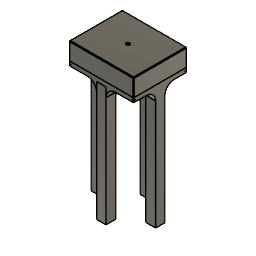
sensing_box (アセンブリ) (Autodesk Fusion 360 archive; units mm, degrees)
design "sensing_box"
Autodesk Fusion 360 part; units mm, degrees
sketch "スケッチ1" plane through (0, 0, 0) normal (0, 0, 1) x (1, 0, 0)
  line L0 (50, 40) -> (-50, 40)
  line L1 (-50, 40) -> (-50, -40)
  line L2 (-50, -40) -> (50, -40)
  line L3 (50, -40) -> (50, 40)
  line L4 (50, 40) -> (-50, -40) construction
  line L5 (-50, 40) -> (50, -40) construction
  line L6 (-46, 27.5) -> (20.5, 27.5)
  line L7 (20.5, 27.5) -> (20.5, -27.5)
  line L8 (20.5, -27.5) -> (-46, -27.5)
  line L9 (-46, -27.5) -> (-46, 27.5)
  line L10 (-46, 27.5) -> (20.5, -27.5) construction
  line L11 (20.5, 27.5) -> (-46, -27.5) construction
  line L12 (-50, 0) -> (-46, 0)
  line L13 (-46, 27.5) -> (-43.75, 27.5)
  line L14 (-43.75, 27.5) -> (-43.75, 25.25)
  line L15 (-43.75, 25.25) -> (-46, 25.25)
  line L16 (-46, 25.25) -> (-46, 27.5)
  line L17 (20, 0) -> (2.5, 0)
  line L18 (-43.75, -27.5) -> (-43.75, -25.25)
  line L19 (-43.75, -25.25) -> (-46, -25.25)
  line L20 (-12.75, 27.5) -> (-12.75, 25)
  line L21 (18.25, 25.25) -> (20.5, 25.25)
  line L22 (18.25, 27.5) -> (18.25, 25.25)
  line L23 (18.25, -25.25) -> (20.5, -25.25)
  line L24 (18.25, -27.5) -> (18.25, -25.25)
  line L25 (47.5, 27) -> (23.5, 27)
  line L26 (23.5, 27) -> (23.5, -27)
  line L27 (23.5, -27) -> (47.5, -27)
  line L28 (47.5, -27) -> (47.5, 27)
  line L29 (47.5, 27) -> (23.5, -27) construction
  line L30 (23.5, 27) -> (47.5, -27) construction
  line L31 (20.5, 0) -> (23.5, 0)
  line L32 (47.5, 27) -> (45, 27)
  line L33 (45, 27) -> (45, 18)
  line L34 (45, 18) -> (47.5, 18)
  line L35 (47.5, 18) -> (47.5, 27)
  line L36 (23.5, -27) -> (26, -27)
  line L37 (26, -27) -> (26, -18)
  line L38 (26, -18) -> (23.5, -18)
  line L39 (23.5, -18) -> (23.5, -27)
  point P0 (-12.75, 0)
  point P1 (35.5, 0)
  dimension "d1" = 100
  dimension "d2" = 80
  dimension "d3" = 66.5
  dimension "d4" = 55
  dimension "d5" = 4
  dimension "d6" = 2.25
  dimension "d7" = 2.25
  dimension "d8" = 24
  dimension "d9" = 54
  dimension "d10" = 3
  dimension "d13" = 2.5
  dimension "d14" = 9
  dimension "d15" = 2.5
  dimension "d16" = 9
  constraint horizontal L0
  constraint perpendicular L0 L1
  constraint parallel L0 L2
  constraint parallel L1 L3
  constraint coincident L4 origin
  constraint coincident L5 origin
  constraint horizontal L6
  constraint perpendicular L6 L7
  constraint parallel L6 L8
  constraint parallel L7 L9
  constraint coincident L10 P0
  constraint coincident L11 P0
  constraint midpoint L1 L12.start
  constraint midpoint L9 L12.end
  constraint perpendicular L9 L12
  constraint horizontal L13
  constraint vertical L14
  constraint horizontal L15
  constraint vertical L16
  constraint symmetric L13.end L17 L18.start
  constraint symmetric L14.end L17 L18.end
  constraint symmetric L15.end L17 L19.end
  constraint midpoint L6 L20.start
  constraint perpendicular L6 L20
  constraint symmetric L13.end L20 L22.start
  constraint symmetric L14.end L20 L21.start
  constraint symmetric L15.end L20 L21.end
  constraint symmetric L18.start L20 L24.start
  constraint symmetric L18.end L20 L23.start
  constraint symmetric L19.end L20 L23.end
  constraint horizontal L25
  constraint perpendicular L25 L26
  constraint parallel L25 L27
  constraint parallel L26 L28
  constraint coincident L29 P1
  constraint coincident L30 P1
  constraint midpoint L7 L31.start
  constraint midpoint L26 L31.end
  constraint horizontal L32
  constraint vertical L33
  constraint horizontal L34
  constraint vertical L35
  constraint horizontal L36
  constraint vertical L37
  constraint horizontal L38
  constraint vertical L39
  measures "d1" distance of L1.end L2.end
  measures "d2" distance of L0.end L1.end
  measures "d3" distance of L7.end L8.end
  measures "d4" distance of L6.end L7.end
  measures "d5" distance of L12.start L12.end
  measures "d6" distance of L6.start L13.end
  measures "d7" distance of L6.start L15.end
  measures "d8" distance of L26.end L27.end
  measures "d9" distance of L25.end L26.end
  measures "d10" distance of L31.start L31.end
  measures "d13" distance of L25.start L32.end
  measures "d14" distance of L25.start L34.end
  measures "d15" distance of L26.end L36.end
  measures "d16" distance of L26.end L38.end
extrude "押し出し1" add sketch "スケッチ1" along normal blind 5 makes body 1
extrude "押し出し2" add sketch "スケッチ1" along normal blind 3.5 contours L6 L9 L13 L14 L15 L16 | L6 L7 L8 L9 L14 L15 L18 L19 L21 L22 L23 L24 | L6 L7 L21 L22 | L8 L9 L18 L19 | L7 L8 L23 L24 | L25 L28 L32 L33 L34 L35 | L25 L26 L27 L28 L33 L34 L37 L38 | L26 L27 L36 L37 L38 L39 bodies 1
extrude "押し出し3" add sketch "スケッチ1" against normal blind 2 contours L0 L1 L2 L3 | L6 L9 L13 L14 L15 L16 | L6 L7 L8 L9 L14 L15 L18 L19 L21 L22 L23 L24 | L6 L7 L21 L22 | L8 L9 L18 L19 | L7 L8 L23 L24 | L25 L28 L32 L33 L34 L35 | L25 L26 L27 L28 L33 L34 L37 L38 | L26 L27 L36 L37 L38 L39 bodies 1
sketch "スケッチ2" plane through (0, 0, 3.5) normal (0, 0, 1) x (-1, 0, 0)
  line L0 (-23.5, -27) -> (-23.5, 27)
  line L1 (-23.5, 27) -> (-47.5, 27)
  line L2 (-47.5, 27) -> (-47.5, -27)
  line L3 (-47.5, -27) -> (-23.5, -27)
  line L4 (-47.5, -27) -> (-45, -27)
  line L5 (-45, -27) -> (-45, -17.5)
  line L6 (-45, -17.5) -> (-47.5, -17.5)
  line L7 (-47.5, -17.5) -> (-47.5, -27)
  line L8 (-26, 16.5) -> (-23.5, 16.5)
  line L9 (-23.5, 16.5) -> (-23.5, 27)
  line L10 (-23.5, 27) -> (-26, 27)
  line L11 (-26, 27) -> (-26, 16.5)
  dimension "d90" = 10.5
  dimension "d103" = 9.5
  dimension "d104" = 2.5
  dimension "d105" = 2.5
  constraint horizontal L4
  constraint vertical L5
  constraint horizontal L6
  constraint vertical L7
  constraint coincident L2.end L3.start
  constraint horizontal L8
  constraint vertical L9
  constraint horizontal L10
  constraint vertical L11
  constraint coincident L0.end L1.start
  measures "d90" distance of L8.start L10.end
  measures "d103" distance of L4.end L5.end
  measures "d104" distance of L5.end L6.end
  measures "d105" distance of L8.start L8.end
sketch "スケッチ3" plane through (0, 0, 3.5) normal (0, 0, 1) x (-1, 0, 0)
  line L0 (46, -27.5) -> (46, 27.5)
  line L1 (46, 27.5) -> (-20.5, 27.5)
  line L2 (-20.5, 27.5) -> (-20.5, -27.5)
  line L3 (-20.5, -27.5) -> (46, -27.5)
  line L4 (-20.5, 27.5) -> (-17.75, 27.5)
  line L5 (-17.75, 27.5) -> (-17.75, 24.75)
  line L6 (-17.75, 24.75) -> (-20.5, 24.75)
  line L7 (-20.5, 24.75) -> (-20.5, 27.5)
  line L8 (46, 27.5) -> (43.25, 27.5)
  line L9 (43.25, 27.5) -> (43.25, 24.75)
  line L10 (43.25, 24.75) -> (46, 24.75)
  line L11 (46, 24.75) -> (46, 27.5)
  line L12 (-20, 0) -> (-2.5, 0)
  line L13 (-17.75, -24.75) -> (-20.5, -24.75)
  line L14 (-17.75, -27.5) -> (-17.75, -24.75)
  line L15 (43.25, -27.5) -> (43.25, -24.75)
  line L16 (43.25, -24.75) -> (46, -24.75)
  dimension "d21" = 2.75
  dimension "d22" = 2.75
  dimension "d23" = 2.75
  dimension "d24" = 2.75
  constraint horizontal L4
  constraint vertical L5
  constraint horizontal L6
  constraint vertical L7
  constraint coincident L1.end L2.start
  constraint horizontal L8
  constraint vertical L9
  constraint horizontal L10
  constraint vertical L11
  constraint coincident L0.end L1.start
  constraint symmetric L4.end L12 L14.start
  constraint symmetric L5.end L12 L13.start
  constraint symmetric L6.end L12 L13.end
  constraint symmetric L8.end L12 L15.start
  constraint symmetric L9.end L12 L15.end
  constraint symmetric L10.end L12 L16.end
  measures "d21" distance of L1.end L4.end
  measures "d22" distance of L1.end L6.end
  measures "d23" distance of L0.end L8.end
  measures "d24" distance of L0.end L10.end
hole "穴1" at (45, 17.5, 3.5) at (26, -16.5, 3.5) at (17.75, 24.75, 3.5) at (17.75, -24.75, 3.5) at (-43.25, 24.75, 3.5) at (-43.25, -24.75, 3.5) direction (0, 0, -1) diameter 2.529 depth 5 tip angle 180 bodies 1
thread "ねじ1" "ISO Metric profile 3.0 M3x0.5 M3x0.5 6H" thread offset 0 thread depth 7.4
sketch "スケッチ4" plane through (0, 0, 5) normal (0, 0, 1) x (-1, 0, 0)
  line L0 (46, 27.5) -> (46, -27.5)
  line L1 (46, -27.5) -> (-20.5, -27.5)
  line L2 (-20.5, -27.5) -> (-20.5, 27.5)
  line L3 (-20.5, 27.5) -> (46, 27.5)
  line L4 (-47.5, -27) -> (-47.5, 27)
  line L5 (-47.5, 27) -> (-23.5, 27)
  line L6 (-23.5, 27) -> (-23.5, -27)
  line L7 (-23.5, -27) -> (-47.5, -27)
  line L8 (-50, 40) -> (-50, -40)
  line L9 (-50, -40) -> (50, -40)
  line L10 (50, -40) -> (50, 40)
  line L11 (50, 40) -> (-50, 40)
  circle A0 centre (-19.9469, -38.0053) radius 4.5
  line L12 (32.5531, -28.2121) -> (7.5531, -28.2121)
  line L13 (7.5531, -28.2121) -> (7.5531, -47.7121)
  line L14 (7.5531, -47.7121) -> (32.5531, -47.7121)
  line L15 (32.5531, -47.7121) -> (32.5531, -28.2121)
  line L16 (32.5531, -28.2121) -> (7.5531, -47.7121) construction
  line L17 (7.5531, -28.2121) -> (32.5531, -47.7121) construction
  line L18 (32.5531, -28.2121) -> (7.5531, -28.2121)
  line L19 (7.5531, -28.2121) -> (7.5531, -31.2121)
  line L20 (7.5531, -31.2121) -> (32.5531, -31.2121)
  line L21 (32.5531, -31.2121) -> (32.5531, -28.2121)
  line L22 (32.5531, -47.7121) -> (30.0531, -47.7121)
  line L23 (30.0531, -47.7121) -> (30.0531, -45.2121)
  line L24 (30.0531, -45.2121) -> (32.5531, -45.2121)
  line L25 (32.5531, -45.2121) -> (32.5531, -47.7121)
  line L26 (20.0531, -37.9621) -> (0.0531, -37.9621)
  line L27 (0.0531, -37.9621) -> (-19.9469, -38.0053)
  line L28 (20.0531, -47.7121) -> (20.0531, -43)
  line L29 (10.0531, -47.7121) -> (10.0531, -45.2121)
  line L30 (10.0531, -45.2121) -> (7.5531, -45.2121)
  point P0 (20.0531, -37.9621)
  dimension "d30" = 9
  dimension "d31" = 25
  dimension "d32" = 19.5
  dimension "d33" = 3
  dimension "d34" = 2.5
  dimension "d35" = 2.5
  dimension "d40" = 20
  dimension "d41" = 20
  constraint horizontal L12
  constraint perpendicular L12 L13
  constraint parallel L12 L14
  constraint parallel L13 L15
  constraint coincident L16 P0
  constraint coincident L17 P0
  constraint horizontal L18
  constraint vertical L19
  constraint horizontal L20
  constraint vertical L21
  constraint coincident L13 L19.end
  constraint horizontal L22
  constraint vertical L23
  constraint horizontal L24
  constraint vertical L25
  constraint coincident P0 L26.start
  constraint perpendicular L13 L26
  constraint coincident A0.centre L27.end
  constraint midpoint L14 L28.start
  constraint perpendicular L14 L28
  constraint symmetric L22.end L28 L29.start
  constraint symmetric L23.end L28 L29.end
  constraint symmetric L24.end L28 L30.end
  measures "d30" diameter of A0
  measures "d31" distance of L13.end L14.end
  measures "d32" distance of L12.end L13.end
  measures "d33" distance of L12.start L20.end
  measures "d34" distance of L14.end L22.end
  measures "d35" distance of L14.end L24.end
  measures "d40" distance of P0 L26.end
  measures "d41" horizontal distance of L26.end A0.centre
extrude "押し出し4" cut 1 faces at (16.6667, -40, 0.3333) along direction (0, 1, 0) blind 8.25 on bodies 1 bodies 1
extrude "押し出し5" add 1 faces at (16.6667, 40, 2.6667) along direction (0, 1, 0) blind 10.25 on bodies 1 bodies 1
extrude "押し出し6" cut sketch "スケッチ4" against normal blind 7 contours L9 A0 | L9 A0 | L12 L13 L15 L18 L19 L20 L21 bodies 1
extrude "押し出し7" cut sketch "スケッチ4" along normal blind 2 from surface at -7 contours L9 L13 L14 L15 L23 L24 L29 L30 | L9 L13 L15 L20 | L14 L15 L22 L23 L24 L25 | L13 L14 L29 L30 bodies 1
hole "穴2" at (-10.0531, 45.2121, 5) direction (0, 0, -1) diameter 2.529 end up to surface (7 mm away) bodies 1
thread "ねじ2" "ISO Metric profile 3.0 M3x0.5 M3x0.5 6H" major diameter 3.086 minor diameter 2.529 pitch 0.5 angle 60 resizes the face on face at (-11.3172, 45.2436, 3.3333) on bodies 1
extrude "押し出し8" add 1 faces at (16.6667, 50.25, 2.6667) along direction (0, 1, 0) blind 2 on bodies 1 bodies 1
extrude "押し出し9" add 1 faces at (-50, 24.25, 0.3333) along direction (-1, 0, 0) blind 2 on bodies 1 bodies 1
extrude "押し出し10" add 1 faces at (16, -31.75, 2.6667) along direction (0, -1, 0) blind 2 on bodies 1 bodies 1
extrude "押し出し11" add 1 faces at (50, -5.0833, 2.6667) along direction (1, 0, 0) blind 2 on bodies 1 bodies 1
sketch "スケッチ5" plane through (0, 0, 5) normal (0, 0, 1) x (-1, 0, 0)
  line L0 (7.5531, -28.2121) -> (32.5531, -28.2121)
  line L1 (32.5531, -28.2121) -> (32.5531, -31.2121)
  line L2 (32.5531, -31.2121) -> (7.5531, -31.2121)
  line L3 (7.5531, -31.2121) -> (7.5531, -28.2121)
  circle A0 centre (-19.9469, -38.0053) radius 4.5
  line L4 (-52, -52.25) -> (52, -52.25)
  line L5 (52, -52.25) -> (52, 33.75)
  line L6 (52, 33.75) -> (-52, 33.75)
  line L7 (-52, 33.75) -> (-52, -52.25)
  line L8 (46, 27.5) -> (46, -27.5)
  line L9 (46, -27.5) -> (-20.5, -27.5)
  line L10 (-20.5, -27.5) -> (-20.5, 27.5)
  line L11 (-20.5, 27.5) -> (46, 27.5)
  line L12 (-47.5, -27) -> (-47.5, 27)
  line L13 (-47.5, 27) -> (-23.5, 27)
  line L14 (-23.5, 27) -> (-23.5, -27)
  line L15 (-23.5, -27) -> (-47.5, -27)
  line L16 (-47, 28.75) -> (47, 28.75)
  line L17 (47, 28.75) -> (47, -47.25)
  line L18 (47, -47.25) -> (-47, -47.25)
  line L19 (-47, -47.25) -> (-47, 28.75)
  line L20 (-47, 28.75) -> (47, -47.25) construction
  line L21 (47, 28.75) -> (-47, -47.25) construction
  circle A1 centre (10.0531, -45.2121) radius 1.2645
  point P0 (0, -9.25)
  dimension "d59" = 94
  dimension "d60" = 76
  constraint horizontal L16
  constraint perpendicular L16 L17
  constraint parallel L16 L18
  constraint parallel L17 L19
  constraint coincident L20 P0
  constraint coincident L21 P0
  measures "d59" distance of L17.end L18.end
  measures "d60" distance of L16.end L17.end
extrude "押し出し12" add sketch "スケッチ5" along normal blind 25 contours L4 L5 L6 L7 | L12 L13 L15 L19 bodies 1
sketch "スケッチ6" plane through (0, 0, -2) normal (0, 0, -1) x (1, 0, 0)
  line L0 (-52, 33.75) -> (-52, -52.25)
  line L1 (-52, -52.25) -> (52, -52.25)
  line L2 (52, -52.25) -> (52, 33.75)
  line L3 (52, 33.75) -> (-52, 33.75)
  circle A0 centre (19.9469, -38.0053) radius 4.5
  line L4 (-7.5531, -28.2121) -> (-7.5531, -47.7121)
  line L5 (-7.5531, -47.7121) -> (-32.5531, -47.7121)
  line L6 (-32.5531, -47.7121) -> (-32.5531, -28.2121)
  line L7 (-32.5531, -28.2121) -> (-7.5531, -28.2121)
  line L8 (-52, 33.75) -> (-49, 33.75)
  line L9 (-49, 33.75) -> (-49, 30.75)
  line L10 (-49, 30.75) -> (-52, 30.75)
  line L11 (-52, 30.75) -> (-52, 33.75)
  line L12 (-52, -52.25) -> (-49, -52.25)
  line L13 (-49, -52.25) -> (-49, -49.25)
  line L14 (-49, -49.25) -> (-52, -49.25)
  line L15 (-52, -49.25) -> (-52, -52.25)
  line L16 (0, -1.75) -> (0, -22.5)
  line L17 (49, 30.75) -> (52, 30.75)
  line L18 (49, 33.75) -> (49, 30.75)
  line L19 (49, -49.25) -> (52, -49.25)
  line L20 (49, -52.25) -> (49, -49.25)
  dimension "d63" = 3
  dimension "d64" = 3
  dimension "d65" = 3
  dimension "d66" = 3
  constraint horizontal L8
  constraint vertical L9
  constraint horizontal L10
  constraint vertical L11
  constraint coincident L0.start L3.end
  constraint horizontal L12
  constraint vertical L13
  constraint horizontal L14
  constraint vertical L15
  constraint coincident L0.end L1.start
  constraint symmetric L8.end L16 L18.start
  constraint symmetric L9.end L16 L17.start
  constraint symmetric L10.end L16 L17.end
  constraint symmetric L12.end L16 L20.start
  constraint symmetric L13.end L16 L19.start
  constraint symmetric L14.end L16 L19.end
  measures "d63" distance of L0.start L8.end
  measures "d64" distance of L0.start L10.end
  measures "d65" distance of L0.end L12.end
  measures "d66" distance of L0.end L14.end
hole "穴3" at (-49, -30.75, -2) at (49, -30.75, -2) at (49, 49.25, -2) at (-49, 49.25, -2) direction (0, 0, 1) diameter 2.93 depth 15 tip angle 180 counterbore diameter 5 counterbore depth 3 bodies 1
thread "ねじ3" "ISO Metric profile 3.5 M3.5x0.6 M3.5x0.6 6H" major diameter 3.5995 minor diameter 2.93 pitch 0.6 angle 60 resizes the face on face at (-47.9016, 48.2806, 5) on face at (48.2994, -32.0366, 5) on face at (-49.7006, -32.0366, 5) on face at (50.0984, 48.2806, 5) on bodies 1
ref_plane "作業平面1" through (0, 9.25, 5) normal (0, 0, 1) x (1, 0, 0)
split "分割1" by plane through (0, 9.25, 5) normal (0, 0, 1) bodies 1 makes body 2 at (-17.3333, -33.75, 13.3333)
sketch "スケッチ7" plane through (0, 0, 30) normal (0, 0, 1) x (-1, 0, 0)
  line L0 (47, -47.25) -> (-47, -47.25)
  line L1 (-47, -47.25) -> (-47, 28.75)
  line L2 (-47, 28.75) -> (47, 28.75)
  line L3 (47, 28.75) -> (47, -47.25)
  line L4 (-52, 33.75) -> (-52, -52.25)
  line L5 (-52, -52.25) -> (52, -52.25)
  line L6 (52, -52.25) -> (52, 33.75)
  line L7 (52, 33.75) -> (-52, 33.75)
  line L8 (52, -52.25) -> (-52, -52.25)
  line L9 (-52, -52.25) -> (-52, 33.75)
  line L10 (-52, 33.75) -> (52, 33.75)
  line L11 (52, 33.75) -> (52, -52.25)
  constraint horizontal L8
  constraint vertical L9
  constraint horizontal L10
  constraint vertical L11
  constraint coincident L4.start L7.end
  constraint coincident L5.end L6.start
extrude "押し出し13" add sketch "スケッチ7" along normal blind 3 contours L0 L1 L2 L3 | L4 L5 L6 L7 L8 L9 L10 L11 bodies 2
sketch "スケッチ8" plane through (0, 0, 33) normal (0, 0, 1) x (-1, 0, 0)
  line L0 (52, 33.75) -> (-52, 33.75)
  line L1 (-52, 33.75) -> (-52, -52.25)
  line L2 (-52, -52.25) -> (52, -52.25)
  line L3 (52, -52.25) -> (52, 33.75)
  line L4 (52, -9.25) -> (-52, -9.25)
  ellipse E0 centre (0, -9.25) end of major axis (3, -9.25) minor radius 2.5
  line L5 (-3, -9.25) -> (3, -9.25) construction
  line L6 (0, -11.75) -> (0, -6.75) construction
  circle A0 centre (-1.5, -9.25) radius 0.75
  circle A1 centre (1.5, -9.25) radius 0.75
  dimension "d77" = 6
  dimension "d78" = 5
  dimension "d93" = 1.5
  dimension "d94" = 1.5
  dimension "d95" = 1.5
  dimension "d96" = 1.5
  constraint midpoint L3 L4.start
  constraint midpoint L1 L4.end
  constraint coincident E0 L5.start
  constraint coincident E0 L5.end
  constraint coincident E0 L6.start
  constraint coincident E0 L6.end
  constraint midpoint L4 E0.centre
  constraint perpendicular L3 L5
  constraint coincident L5 A0.centre
  constraint coincident L5 A1.centre
  measures "d77" distance of E0
  measures "d93" diameter of A0
  measures "d94" diameter of A1
  measures "d95" distance of E0.centre A0.centre
  measures "d96" distance of E0.centre A1.centre
extrude "押し出し14" cut sketch "スケッチ8" against normal blind 2 contours L4 E0 A0 A1 | L4 E0 A0 A1 | L4 A1 | L4 A1 | L4 A0 | L4 A0 bodies 2
sketch "スケッチ9" plane through (0, 52.25, 0) normal (0, 1, 0) x (-1, 0, 0)
  line L0 (-52, 5) -> (52, 5)
  line L1 (52, 5) -> (52, 33)
  line L2 (52, 33) -> (-52, 33)
  line L3 (-52, 33) -> (-52, 5)
  line L4 (-20.5, 31) -> (20.5, 31)
  line L5 (20.5, 31) -> (20.5, 15)
  line L6 (20.5, 15) -> (-20.5, 15)
  line L7 (-20.5, 15) -> (-20.5, 31)
  line L8 (-20.5, 31) -> (20.5, 15) construction
  line L9 (20.5, 31) -> (-20.5, 15) construction
  point P0 (0, 23)
  dimension "d84" = 41
  dimension "d85" = 16
  dimension "d86" = 10
  constraint horizontal L4
  constraint perpendicular L4 L5
  constraint parallel L4 L6
  constraint parallel L5 L7
  constraint coincident L8 P0
  constraint coincident L9 P0
  constraint vertical origin P0
  measures "d84" distance of L5.end L6.end
  measures "d85" distance of L4.end L5.end
  measures "d86" distance of L2 P0
extrude "押し出し15" cut sketch "スケッチ9" against normal up to surface (5 mm away) contours L4 L5 L6 L7 bodies 2
extrude "押し出し16" cut 1 faces at (-2.9129, -7.9872, 3.5) along direction (0, 0, -1) blind 1.5 on bodies 1 bodies 1
extrude "押し出し17" cut sketch "スケッチ8" against normal up to surface (3 mm away) contours L4 A1 | L4 A1 | L4 A0 | L4 A0 bodies 2
fillet "フィレット1" radius 1 8 edges at (52, -33.75, 1.5) (52, 9.25, -2) (52, 52.25, 1.5) (0, 52.25, -2) (-52, 52.25, 1.5) (-52, -33.75, 1.5) (-52, 9.25, -2) (0, -33.75, -2) on bodies 1
fillet "フィレット2" radius 1 8 edges at (52, -33.75, 19) (52, 9.25, 33) (0, -33.75, 33) (-52, 9.25, 33) (-52, -33.75, 19) (0, 52.25, 33) (-52, 52.25, 19) (52, 52.25, 19) on bodies 2
sketch "スケッチ10" plane through (0, 0, -2) normal (0, 0, -1) x (1, 0, 0)
  line L0 (-51, 29.25) -> (-51, -47.75)
  arc A0 (-47.5, -51.25) -> (-51, -47.75) centre (-49, -49.25) ccw
  line L1 (-47.5, -51.25) -> (47.5, -51.25)
  arc A1 (51, -47.75) -> (47.5, -51.25) centre (49, -49.25) ccw
  line L2 (51, -47.75) -> (51, 29.25)
  arc A2 (47.5, 32.75) -> (51, 29.25) centre (49, 30.75) ccw
  line L3 (47.5, 32.75) -> (-47.5, 32.75)
  arc A3 (-51, 29.25) -> (-47.5, 32.75) centre (-49, 30.75) ccw
  circle A4 centre (19.9469, -38.0053) radius 4.5
  line L4 (-7.5531, -28.2121) -> (-7.5531, -47.7121)
  line L5 (-7.5531, -47.7121) -> (-32.5531, -47.7121)
  line L6 (-32.5531, -47.7121) -> (-32.5531, -28.2121)
  line L7 (-32.5531, -28.2121) -> (-7.5531, -28.2121)
  line L8 (-66, -1.75) -> (-36, -1.75)
  line L9 (-36, -1.75) -> (-36, -16.75)
  line L10 (-36, -16.75) -> (-66, -16.75)
  line L11 (-66, -16.75) -> (-66, -1.75)
  line L12 (-66, -1.75) -> (-36, -16.75) construction
  line L13 (-36, -1.75) -> (-66, -16.75) construction
  line L14 (0, -1.75) -> (0, -22.5)
  line L15 (36, -16.75) -> (66, -16.75)
  line L16 (66, -1.75) -> (36, -1.75)
  line L17 (36, -1.75) -> (36, -16.75)
  line L18 (66, -16.75) -> (66, -1.75)
  line L19 (-51, -9.25) -> (-42.6571, -9.25)
  line L20 (7.5, 47.75) -> (-7.5, 47.75)
  line L21 (-7.5, 47.75) -> (-7.5, 17.75)
  line L22 (-7.5, 17.75) -> (7.5, 17.75)
  line L23 (7.5, 17.75) -> (7.5, 47.75)
  line L24 (7.5, 47.75) -> (-7.5, 17.75) construction
  line L25 (-7.5, 47.75) -> (7.5, 17.75) construction
  line L26 (-7.5, -66.25) -> (-7.5, -36.25)
  line L27 (7.5, -66.25) -> (-7.5, -66.25)
  line L28 (7.5, -36.25) -> (7.5, -66.25)
  line L29 (-7.5, -36.25) -> (7.5, -36.25)
  line L30 (52, -52.2245) -> (-52, -52.2245)
  line L31 (-52, -52.2245) -> (-52, 33.7755)
  line L32 (-52, 33.7755) -> (52, 33.7755)
  line L33 (52, 33.7755) -> (52, -52.2245)
  line L34 (52, -52.2245) -> (-52, 33.7755) construction
  line L35 (-52, -52.2245) -> (52, 33.7755) construction
  point P0 (-51, -9.25)
  point P1 (0, 32.75)
  point P2 (0, -9.2245)
  dimension "d106" = 30
  dimension "d107" = 15
  dimension "d108" = 15
  dimension "d109" = 30
  dimension "d112" = 104
  dimension "d113" = 86
  constraint horizontal L8
  constraint perpendicular L8 L9
  constraint parallel L8 L10
  constraint parallel L9 L11
  constraint coincident L12 P0
  constraint coincident L13 P0
  constraint midpoint L0 P0
  constraint symmetric L8.start L14 L16.start
  constraint symmetric L8.end L14 L16.end
  constraint symmetric L9.end L14 L15.start
  constraint symmetric L10.end L14 L15.end
  constraint coincident P0 L19.start
  constraint perpendicular L0 L19
  constraint horizontal L20
  constraint perpendicular L20 L21
  constraint parallel L20 L22
  constraint parallel L21 L23
  constraint coincident L24 P1
  constraint coincident L25 P1
  constraint midpoint L3 P1
  constraint symmetric L19 L20.start L27.start
  constraint symmetric L19 L20.end L26.start
  constraint symmetric L19 L21.end L26.end
  constraint symmetric L19 L22.end L28.start
  constraint horizontal L30
  constraint perpendicular L30 L31
  constraint parallel L30 L32
  constraint parallel L31 L33
  constraint coincident L34 P2
  constraint coincident L35 P2
  constraint coincident L14 P2
  measures "d106" distance of L9.end L10.end
  measures "d107" distance of L8.end L9.end
  measures "d108" distance of L21.end L22.end
  measures "d109" distance of L20.end L21.end
  measures "d112" distance of L31.end L32.end
  measures "d113" distance of L30.end L31.end
extrude "押し出し18" add sketch "スケッチ10" along normal blind 200 contours L0 L8 L9 L10 | L0 L8 L10 L31 | L3 L21 L23 L32 | L3 L21 L22 L23 | L1 L26 L28 L30 | L1 L26 L28 L29 | L2 L15 L16 L33 | L2 L15 L16 L17 bodies 1
delete_face "面を削除1" 1 faces at (51.1305, -33.5776, -1.5459) on bodies 1
delete_face "面を削除2" 1 faces at (51.1305, 52.0776, -1.5459) on bodies 1
delete_face "面を削除3" 1 faces at (-51.8276, 51.7959, -1.1305) on bodies 1
delete_face "面を削除4" 1 faces at (-51.8276, -32.8805, -1.5459) on bodies 1
delete_face "面を削除5" 1 faces at (-51.9877, -4.75, -1.1564) on bodies 1
delete_face "面を削除6" 1 faces at (17, -33.7414, -1.1305) on bodies 1
delete_face "面を削除7" 1 faces at (17, 52.2414, -1.1305) on bodies 1
delete_face "面を削除8" 1 faces at (51.8708, -4.8731, -1.4916) on bodies 1
fillet "フィレット3" radius 15 12 edges at (-44, 1.75, -2) (-36, 9.25, -2) (-44, 16.75, -2) (-7.5, -25.75, -2) (0, -17.75, -2) (7.5, -25.75, -2) (0, 36.25, -2) (7.5, 44.2373, -2) (-7.5, 44.2373, -2) (44, 1.75, -2) (36, 9.25, -2) (44, 16.75, -2) on bodies 1
chamfer "面取り1" distance 7.5 angle 45 16 edges at (0, -33.7755, -202) (-7.5, -25.7627, -202) (7.5, -25.7627, -202) (0, -17.75, -202) (-36, 9.25, -202) (-44, 1.75, -202) (-52, 9.25, -202) (-44, 16.75, -202) (-7.5, 44.2373, -202) (0, 36.25, -202) (7.5, 44.2373, -202) (0, 52.2245, -202) (36, 9.25, -202) (44, 1.75, -202) (52, 9.25, -202) (44, 16.75, -202) on bodies 1
